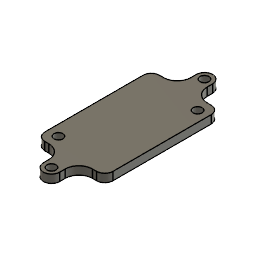
Voltage Booster Mount (Autodesk Fusion 360 design; units mm, degrees)
part number: 2026-05-14-16-24-24-619
Autodesk Fusion 360 part; units mm, degrees
note: some values were not read from the file. Set by a fixed rule: which sketch regions a step uses.
sketch "Sketch1" plane through (0, 0, 0) normal (0, 1, 0) x (1, 0, 0)
  line L0 (-12.5, 21) -> (12.5, 21)
  line L1 (12.5, 21) -> (12.5, -21)
  line L2 (12.5, -21) -> (-12.5, -21)
  line L3 (-12.5, -21) -> (-12.5, 21)
  line L4 (-12.5, 21) -> (12.5, -21) construction
  line L5 (12.5, 21) -> (-12.5, -21) construction
  line L6 (-8.625, 16.855) -> (8.625, 16.855) construction
  line L7 (8.625, 16.855) -> (8.625, -16.855) construction
  line L8 (8.625, -16.855) -> (-8.625, -16.855) construction
  line L9 (-8.625, -16.855) -> (-8.625, 16.855) construction
  line L10 (-8.625, 16.855) -> (8.625, -16.855) construction
  line L11 (8.625, 16.855) -> (-8.625, -16.855) construction
  circle A0 centre (8.625, 16.855) radius 1.65
  circle A1 centre (-8.625, -16.855) radius 1.65
  line L12 (0, 0) -> (0, 28) construction
  line L13 (0, 0) -> (0, -28) construction
  circle A2 centre (0, 28) radius 1.65
  line L14 (0, 28) -> (-1.65, 28) construction
  circle A3 centre (0, 28) radius 3
  line L15 (0, 28) -> (-3, 28)
  line L16 (-3, 28) -> (-3, 21)
  line L17 (3, 28) -> (3, 21)
  line L18 (-3, -28) -> (-3, -21)
  circle A4 centre (0, -28) radius 3
  line L19 (3, -28) -> (3, -21)
  circle A5 centre (0, -28) radius 1.65
  line L20 (0, 0) -> (12.5, 0) construction
  dimension "d1" = 25
  dimension "d2" = 42
  dimension "d3" = 17.25
  dimension "d4" = 33.71
  dimension "d9" = 3.3
  dimension "d10" = 3.3
  dimension "d13" = 28
  dimension "d14" = 28
  dimension "d15" = 3.3
  dimension "d17" = 6
  constraint horizontal L0
  constraint perpendicular L0 L1
  constraint parallel L0 L2
  constraint parallel L1 L3
  constraint coincident L4 L12.start
  constraint coincident L5 L12.start
  constraint coincident L12.start L13.start
  constraint horizontal L6
  constraint perpendicular L6 L7
  constraint parallel L6 L8
  constraint parallel L7 L9
  constraint coincident L10 L12.start
  constraint coincident L11 L12.start
  constraint coincident L6.end L7.start
  constraint coincident L8.end L9.start
  constraint vertical L12
  constraint vertical L13
  constraint coincident L12.end A2.centre
  constraint coincident A2 L14.end
  constraint perpendicular L12 L14
  constraint concentric A2 A3
  constraint coincident A3 L15.end
  constraint perpendicular L12 L15
  constraint coincident L0 L16.end
  constraint tangent A3 L16
  constraint coincident A3 L17.start
  constraint coincident L0 L17.end
  constraint tangent A3 L17
  constraint perpendicular L0 L17
  measures "d1" distance of L1.end L2.end
  measures "d2" distance of L0.end L1.end
  measures "d3" distance of L7.end L8.end
  measures "d4" distance of L6.end L7.end
  measures "d9" diameter of A0
  measures "d10" diameter of A1
  measures "d13" distance of L12.start L12.end
  measures "d14" distance of L12.start L13.end
  measures "d15" diameter of A2
  measures "d17" diameter of A3
extrude "Extrude2" add sketch "Sketch1" along normal blind 3
fillet "Fillet2" radius 3 4 edges at (12.5, 1.5, 21) (-12.5, 1.5, 21) (12.5, 1.5, -21) (-12.5, 1.5, -21)
fillet "Fillet3" radius 5 4 edges at (3, 1.5, 21) (-3, 1.5, 21) (-3, 1.5, -21) (3, 1.5, -21)
